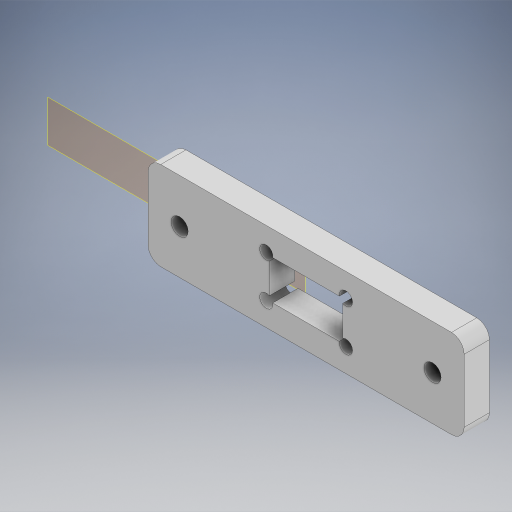
# Autodesk Inventor part: front of head(under)_zig6
Saved by Autodesk Inventor 2024 (Build 280153000, 153)
## iProperties
Created: 2024-09-11
Part Number: front of head(under)_zig6
Material: 일반
Document SubType Name: Modeling
Designer: ASUS
Density: 1 g/cm^3
Appearance: 기본값
Author: ASUS
Autodesk Inventor part; units mm, degrees
ref_plane "YZ Plane" through (0, 0, 0) normal (1, 0, 0) x (0, 1, 0)
ref_plane "XZ Plane" through (0, 0, 0) normal (0, 1, 0) x (-1, 0, 0)
ref_plane "XY Plane" through (0, 0, 0) normal (0, 0, 1) x (1, 0, 0)
ref_plane "작업 평면1" through (0, 0, 0) normal (0, 0, 1) x (1, 0, 0)
sketch "스케치1" plane through (0, 0, 0) normal (0, 0, 1) x (1, 0, 0)
  line L0 (6, -3) -> (6, 3) projected
  line L1 (6, 3) -> (-6, 3) projected
  line L2 (-6, 3) -> (-6, -3) projected
  line L3 (-6, -3) -> (6, -3) projected
  line L4 (-6.3, 3.3) -> (6.3, 3.3)
  line L5 (6.3, 3.3) -> (6.3, -3.3)
  line L6 (6.3, -3.3) -> (-6.3, -3.3)
  line L7 (-6.3, -3.3) -> (-6.3, 3.3)
  line L8 (-43, 3) -> (43, 3)
  line L9 (43, 3) -> (43, -3)
  line L10 (43, -3) -> (-43, -3)
  line L11 (-43, -3) -> (-43, 3)
  line L12 (47, 7) -> (-47, 7)
  line L13 (-47, 7) -> (-47, -7)
  line L14 (-47, -7) -> (47, -7)
  line L15 (47, -7) -> (47, 7)
  line L16 (-6, -3) -> (-6, 3) projected
  line L17 (-6, 3) -> (-43, 3) projected
  line L18 (-43, -3) -> (-43, 3) projected
  line L19 (-6, -3) -> (-43, -3) projected
  circle A0 centre (-20, 0) radius 1.35 projected
  line L20 (6, 3) -> (6, -3) projected
  line L21 (6, -3) -> (43, -3) projected
  line L22 (43, 3) -> (43, -3) projected
  line L23 (6, 3) -> (43, 3) projected
  circle A1 centre (20, 0) radius 1.35 projected
  line L24 (-25, -7) -> (-15, -7)
  line L25 (-15, -7) -> (-15, 7)
  line L26 (-15, 7) -> (-25, 7)
  line L27 (-25, 7) -> (-25, -7)
  line L28 (-25, -7) -> (-15, 7) construction
  line L29 (-15, -7) -> (-25, 7) construction
  line L30 (15, -7) -> (25, -7)
  line L31 (25, -7) -> (25, 7)
  line L32 (25, 7) -> (15, 7)
  line L33 (15, 7) -> (15, -7)
  line L34 (15, -7) -> (25, 7) construction
  line L35 (25, -7) -> (15, 7) construction
  circle A2 centre (-6.3, 3.3) radius 1.05
  circle A3 centre (6.3, 3.3) radius 1.05
  circle A4 centre (6.3, -3.3) radius 1.05
  circle A5 centre (-6.3, -3.3) radius 1.05
  point P0 (0, 0)
  point P1 (6, 2.2938)
  point P2 (6, -2.2938)
  point P3 (5.25, -3.3)
  point P4 (-5.25, -3.3)
  point P5 (-6, -2.2938)
  point P6 (-6, 2.2938)
  point P7 (-5.25, 3.3)
  point P8 (5.25, 3.3)
  dimension "d0" = 0.3
  dimension "d1" = 4
  dimension "d2" = 10
  dimension "d3" = 14
  dimension "d4" = 10
  dimension "d5" = 14
  dimension "d6" = 2.1
  dimension "d7" = 2.1
  dimension "d8" = 2.1
  dimension "d9" = 2.1
  constraints: 48 end point, 8 parallel, 4 centre point, 4 midpoint, 4 perpendicular, 3 horizontal, 1 coincident, 8 other
  measures "d0" distance between parallel lines of L1 L4
  measures "d1" distance between parallel lines of L8 L12
  measures "d2" distance of L26.end L25.end
  measures "d3" distance of L25.end L24.end
  measures "d4" distance of L32.end L31.end
  measures "d5" distance of L31.end L30.end
  measures "d6" diameter of A2
  measures "d7" diameter of A3
  measures "d8" diameter of A4
  measures "d9" diameter of A5
extrude "돌출1" add sketch "스케치1" along normal blind 4 contours L0 A3 L5 A4 | L5 A3 L8 L33 L10 A4 | A4 L10 L33 L14 L25 A5 L6 | A5 L7 A2 L2 | L33 L8 L31 L10 | L10 L31 L14 L33 | L4 A2 L8 L25 L12 L33 A3 | L10 L25 L8 A2 L7 A5 | L33 L12 L31 L8 | L25 L14 L27 L10 | L10 L27 L8 L25 | L8 L27 L12 L25
fillet "모깎기1" radius 2 4 edges at (-25, -7, 2) (-25, 7, 2) (25, 7, 2) (25, -7, 2)
sketch "스케치2" plane through (0, 0, 4) normal (0, 0, 1) x (1, 0, 0)
  arc A0 (23, -7) -> (25, -5) centre (23, -5) ccw projected
  line L0 (25, -5) -> (25, 5) projected
  arc A1 (25, 5) -> (23, 7) centre (23, 5) ccw projected
  line L1 (23, 7) -> (-23, 7) projected
  arc A2 (-23, 7) -> (-25, 5) centre (-23, 5) ccw projected
  line L2 (-25, 5) -> (-25, -5) projected
  arc A3 (-25, -5) -> (-23, -7) centre (-23, -5) ccw projected
  line L3 (-23, -7) -> (23, -7) projected
  circle A4 centre (20, 0) radius 1.35 projected
  arc A5 (6, 2.2938) -> (5.25, 3.3) centre (6.3, 3.3) ccw projected
  line L4 (6, 2.2938) -> (6, -2.2938) projected
  arc A6 (5.25, -3.3) -> (6, -2.2938) centre (6.3, -3.3) ccw projected
  line L5 (5.25, -3.3) -> (-5.25, -3.3) projected
  arc A7 (-6, -2.2938) -> (-5.25, -3.3) centre (-6.3, -3.3) ccw projected
  line L6 (-6, -2.2938) -> (-6, 2.2938) projected
  arc A8 (-5.25, 3.3) -> (-6, 2.2938) centre (-6.3, 3.3) ccw projected
  line L7 (-5.25, 3.3) -> (5.25, 3.3) projected
  circle A9 centre (-20, 0) radius 1.35 projected
  arc A10 (5.8, 2.6126) -> (5.4739, 3.1) centre (6.3, 3.3) ccw
  line L8 (5.8, 2.6126) -> (5.8, -2.6126)
  arc A11 (5.4739, -3.1) -> (5.8, -2.6126) centre (6.3, -3.3) ccw
  line L9 (5.4739, -3.1) -> (-5.4739, -3.1)
  arc A12 (-5.8, -2.6126) -> (-5.4739, -3.1) centre (-6.3, -3.3) ccw
  line L10 (-5.8, -2.6126) -> (-5.8, 2.6126)
  arc A13 (-5.4739, 3.1) -> (-5.8, 2.6126) centre (-6.3, 3.3) ccw
  line L11 (-5.4739, 3.1) -> (5.4739, 3.1)
  point P0 (0, 0)
  dimension "d13" = 0.2
  constraints: 8 end point, 8 point on circle, 4 centre point, 7 other
  measures "d13" distance between parallel lines of L7 L11
extrude "돌출2" add sketch "스케치2" against normal up to surface (4 mm away) contours L4 A6 L5 A7 L6 A8 L7 A5
sketch "스케치3" plane through (0, 0, 4) normal (0, 0, 1) x (1, 0, 0)
  line L0 (5.4739, -3.1) -> (-5.4739, -3.1) projected
  arc A0 (-5.8, -2.6126) -> (-5.4739, -3.1) centre (-6.3, -3.3) ccw projected
  line L1 (-5.8, -2.6126) -> (-5.8, 2.6126) projected
  arc A1 (-5.4739, 3.1) -> (-5.8, 2.6126) centre (-6.3, 3.3) ccw projected
  line L2 (-5.4739, 3.1) -> (5.4739, 3.1) projected
  arc A2 (5.8, 2.6126) -> (5.4739, 3.1) centre (6.3, 3.3) ccw projected
  line L3 (5.8, 2.6126) -> (5.8, -2.6126) projected
  arc A3 (5.4739, -3.1) -> (5.8, -2.6126) centre (6.3, -3.3) ccw projected
  arc A4 (23, -7) -> (25, -5) centre (23, -5) ccw projected
  line L4 (25, -5) -> (25, 5) projected
  arc A5 (25, 5) -> (23, 7) centre (23, 5) ccw projected
  line L5 (23, 7) -> (-23, 7) projected
  arc A6 (-23, 7) -> (-25, 5) centre (-23, 5) ccw projected
  line L6 (-25, 5) -> (-25, -5) projected
  arc A7 (-25, -5) -> (-23, -7) centre (-23, -5) ccw projected
  line L7 (-23, -7) -> (23, -7) projected
  circle A8 centre (20, 0) radius 1.35 projected
  circle A9 centre (-20, 0) radius 1.35 projected
  point P0 (0, 0)
hole "구멍1" at (-6.3, 3.3, 4) at (-6.3, -3.3, 4) at (6.3, -3.3, 4) at (6.3, 3.3, 4) direction (0, 0, -1) diameter 2.1 end through all
